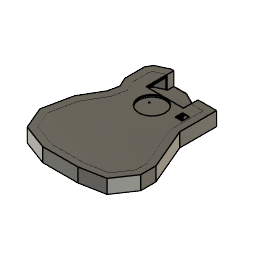
guitar body (Autodesk Fusion 360 design; units mm, degrees)
part number: 2026-05-27-12-41-13-144
Autodesk Fusion 360 part; units mm, degrees
note: some values were not read from the file. Chosen so that the rebuilt part matches the saved one: which bodies a step acts on.
sketch "Sketch1" plane through (0, 0, 0) normal (0, 0, 1) x (1, 0, 0)
  line L0 (251.1628, 0) -> (195.3488, 0)
  line L1 (195.3488, 0) -> (151.6873, -20.8028)
  line L2 (151.6873, -20.8028) -> (139.5523, -41.6057)
  line L3 (139.5523, -41.6057) -> (139.5523, -55.814)
  line L4 (139.5523, -55.814) -> (139.5523, -83.7209)
  line L5 (139.5523, -83.7209) -> (139.5523, -114.4156)
  line L6 (139.5523, -114.4156) -> (155.4368, -147.7543)
  line L7 (155.4368, -147.7543) -> (147.4945, -185.4919)
  line L8 (147.4945, -185.4919) -> (127.7472, -219.3445)
  line L9 (127.7472, -219.3445) -> (103.1629, -261.4891)
  line L10 (103.1629, -261.4891) -> (81.0774, -366.4285)
  line L11 (81.0774, -366.4285) -> (115.455, -447.2608)
  line L12 (115.455, -447.2608) -> (206.2947, -481.0654)
  line L13 (206.2947, -481.0654) -> (334.8837, -481.0654)
  line L14 (334.8837, -481.0654) -> (424.7244, -464.1631)
  line L15 (424.7244, -464.1631) -> (474.4186, -390.6977)
  line L16 (474.4186, -390.6977) -> (474.4186, -334.8837)
  line L17 (474.4186, -334.8837) -> (443.8402, -262.9846)
  line L18 (443.8402, -262.9846) -> (410.1145, -183.6851)
  line L19 (410.1145, -183.6851) -> (410.1145, -83.7209)
  line L20 (410.1145, -83.7209) -> (410.1145, -48.5399)
  line L21 (410.1145, -48.5399) -> (381.3852, -48.5399)
  line L22 (381.3852, -48.5399) -> (334.8837, -48.5399)
  line L23 (334.8837, -48.5399) -> (306.9767, -27.907)
  line L24 (306.9767, -27.907) -> (251.1628, 0)
  constraint horizontal L0
  constraint perpendicular L0 L3
  constraint perpendicular L0 L4
  constraint perpendicular L1 L6
  constraint parallel L2 L8
  constraint parallel L8 L9
  constraint parallel L7 L10
  constraint horizontal L13
  constraint vertical L16
  constraint parallel L11 L17
  constraint parallel L17 L18
  constraint parallel L16 L19
  constraint parallel L19 L20
  constraint perpendicular L20 L21
  constraint perpendicular L20 L22
extrude "Extrude1" add sketch "Sketch1" along normal blind 100 makes body 1
sketch "Sketch2" plane through (0, 0, 100) normal (0, 0, 1) x (-1, 0, 0)
  line L0 (-306.9767, 27.907) -> (-251.1628, 0)
  line L1 (-251.1628, 0) -> (-195.3488, 0)
  line L2 (-195.3488, 0) -> (-151.6873, 20.8028)
  line L3 (-151.6873, 20.8028) -> (-139.5523, 41.6057)
  line L4 (-139.5523, 41.6057) -> (-139.5523, 114.4156)
  line L5 (-139.5523, 114.4156) -> (-155.4368, 147.7543)
  line L6 (-155.4368, 147.7543) -> (-147.4945, 185.4919)
  line L7 (-147.4945, 185.4919) -> (-103.1629, 261.4891)
  line L8 (-103.1629, 261.4891) -> (-81.0774, 366.4285)
  line L9 (-81.0774, 366.4285) -> (-115.455, 447.2608)
  line L10 (-115.455, 447.2608) -> (-206.2947, 481.0654)
  line L11 (-206.2947, 481.0654) -> (-334.8837, 481.0654)
  line L12 (-334.8837, 481.0654) -> (-424.7244, 464.1631)
  line L13 (-424.7244, 464.1631) -> (-474.4186, 390.6977)
  line L14 (-474.4186, 390.6977) -> (-474.4186, 334.8837)
  line L15 (-474.4186, 334.8837) -> (-410.1145, 183.6851)
  line L16 (-410.1145, 183.6851) -> (-410.1145, 48.5399)
  line L17 (-410.1145, 48.5399) -> (-334.8837, 48.5399)
  line L18 (-334.8837, 48.5399) -> (-306.9767, 27.907)
  circle A0 centre (-275, 150) radius 48.1981
extrude "Extrude2" cut sketch "Sketch2" against normal blind 90 contours A0 bodies 1
shell "Shell1" thickness 25 removed faces 1 at (226.8618, -147.5975, 40) on bodies 1
sketch "Sketch3" plane through (0, 0, 25) normal (0, 0, 1) x (-1, 0, 0)
  circle A0 centre (-275, 150) radius 48.1981
  line L0 (-293.8574, 49.2981) -> (-245.2611, 25)
  line L1 (-245.2611, 25) -> (-201.0002, 25)
  line L2 (-201.0002, 25) -> (-169.3983, 40.0569)
  line L3 (-169.3983, 40.0569) -> (-164.5523, 48.3644)
  line L4 (-164.5523, 48.3644) -> (-164.5523, 108.7642)
  line L5 (-164.5523, 108.7642) -> (-181.6416, 144.6317)
  line L6 (-181.6416, 144.6317) -> (-171.126, 194.5966)
  line L7 (-171.126, 194.5966) -> (-126.7944, 270.5938)
  line L8 (-126.7944, 270.5938) -> (-107.1611, 363.8814)
  line L9 (-107.1611, 363.8814) -> (-134.2523, 427.581)
  line L10 (-134.2523, 427.581) -> (-210.7956, 456.0654)
  line L11 (-210.7956, 456.0654) -> (-332.5525, 456.0654)
  line L12 (-332.5525, 456.0654) -> (-409.8575, 441.5215)
  line L13 (-409.8575, 441.5215) -> (-449.4186, 383.0364)
  line L14 (-449.4186, 383.0364) -> (-449.4186, 339.9791)
  line L15 (-449.4186, 339.9791) -> (-385.1145, 188.7805)
  line L16 (-385.1145, 188.7805) -> (-385.1145, 73.5399)
  line L17 (-385.1145, 73.5399) -> (-326.6455, 73.5399)
  line L18 (-326.6455, 73.5399) -> (-293.8574, 49.2981)
extrude "Extrude3" cut sketch "Sketch3" against normal blind 20 bodies 1
sketch "Sketch4" plane through (0, 0, 100) normal (0, 0, 1) x (-1, 0, 0)
  circle A0 centre (-275, 150) radius 48.1981
  line L0 (-306.9767, 27.907) -> (-251.1628, 0)
  line L1 (-251.1628, 0) -> (-195.3488, 0)
  line L2 (-195.3488, 0) -> (-151.6873, 20.8028)
  line L3 (-151.6873, 20.8028) -> (-139.5523, 41.6057)
  line L4 (-139.5523, 41.6057) -> (-139.5523, 114.4156)
  line L5 (-139.5523, 114.4156) -> (-155.4368, 147.7543)
  line L6 (-155.4368, 147.7543) -> (-147.4945, 185.4919)
  line L7 (-147.4945, 185.4919) -> (-103.1629, 261.4891)
  line L8 (-103.1629, 261.4891) -> (-81.0774, 366.4285)
  line L9 (-81.0774, 366.4285) -> (-115.455, 447.2608)
  line L10 (-115.455, 447.2608) -> (-206.2947, 481.0654)
  line L11 (-206.2947, 481.0654) -> (-334.8837, 481.0654)
  line L12 (-334.8837, 481.0654) -> (-424.7244, 464.1631)
  line L13 (-424.7244, 464.1631) -> (-474.4186, 390.6977)
  line L14 (-474.4186, 390.6977) -> (-474.4186, 334.8837)
  line L15 (-474.4186, 334.8837) -> (-410.1145, 183.6851)
  line L16 (-410.1145, 183.6851) -> (-410.1145, 48.5399)
  line L17 (-410.1145, 48.5399) -> (-334.8837, 48.5399)
  line L18 (-334.8837, 48.5399) -> (-306.9767, 27.907)
  line L19 (-205.3595, 101.8019) -> (-341.7535, 101.8019)
  line L20 (-341.7535, 101.8019) -> (-341.7535, -17.2484)
  line L21 (-341.7535, -17.2484) -> (-205.3595, -17.2484)
  line L22 (-205.3595, -17.2484) -> (-205.3595, 101.8019)
  circle A1 centre (-335.8345, 95.8779) radius 2.3
  circle A2 centre (-211.2785, 95.8779) radius 2.3
  dimension "d9" = 136.394
  dimension "d10" = 5.919
  dimension "d11" = 5.924
  dimension "d12" = 4.6
  dimension "d13" = 5.919
  dimension "d14" = 5.924
  dimension "d15" = 4.6
  constraint horizontal L19
  constraint vertical L20
  constraint horizontal L21
  constraint vertical L22
  constraint tangent A0 L19
  measures "d9" distance of L19.start L19.end
  measures "d10" distance of L20 A1.centre
  measures "d11" distance of L19 A1.centre
  measures "d12" diameter of A1
  measures "d13" distance of L22 A2.centre
  measures "d14" distance of L19 A2.centre
  measures "d15" diameter of A2
extrude "Extrude4" cut sketch "Sketch4" against normal blind 95 contours L0 L1 L17 L18 L19 L20 L22 bodies 1 makes body 2 at (213.2984, -94.7779, 83.3333) makes body 3 at (335.102, -98.0582, 91.6667)
extrude "Extrude5" cut 1 faces at (293.8474, -161.9933, 10) along direction (0, 0, -1) blind 5 on bodies 1 bodies 1
extrude "Extrude6" cut 1 faces at (210.9984, -97.2569, 100) along direction (0, 0, -1) blind 170 on bodies 2 bodies 1 2
extrude "Extrude7" cut 1 faces at (335.6639, -96.6254, 100) along direction (0, 0, -1) blind 105 on bodies 3 bodies 1 3
extrude "Extrude8" add 1 faces at (366.8466, -337.1099, 100) along direction (0, 0, -1) blind 47.8 on bodies 1 bodies 1 2 3
extrude "Extrude9" cut 1 faces at (366.8466, -337.1099, 100) along direction (0, 0, -1) blind 40 on bodies 1 bodies 1
extrude "Extrude10" cut 1 faces at (297.4976, -283.4142, 0) along direction (0, 0, 1) blind 4 on bodies 1 bodies 1
extrude "Extrude11" add 1 faces at (355.458, -331.1055, 52.2) along direction (0, 0, -1) blind 5 separate body on bodies 1 makes body 4
extrude "Extrude12" cut 1 faces at (366.8466, -337.1099, 60) along direction (0, 0, -1) blind 5 on bodies 1 bodies 1
sketch "Sketch5" plane through (0, 0, 55) normal (0, 0, 1) x (-1, 0, 0)
  line L0 (-341.7535, 48.5399) -> (-341.7535, 101.8019)
  line L1 (-341.7535, 101.8019) -> (-275, 101.8019)
  circle A0 centre (-275, 150) radius 48.1981
  line L2 (-275, 101.8019) -> (-205.3595, 101.8019)
  line L3 (-205.3595, 101.8019) -> (-205.3595, 0)
  line L4 (-205.3595, 0) -> (-195.3489, 0)
  line L5 (-195.3489, 0) -> (-151.6873, 20.8028)
  line L6 (-151.6873, 20.8028) -> (-139.5523, 41.6057)
  line L7 (-139.5523, 41.6057) -> (-139.5523, 114.4156)
  line L8 (-139.5523, 114.4156) -> (-155.4368, 147.7543)
  line L9 (-155.4368, 147.7543) -> (-147.4946, 185.4919)
  line L10 (-147.4946, 185.4919) -> (-103.1629, 261.4891)
  line L11 (-103.1629, 261.4891) -> (-81.0774, 366.4285)
  line L12 (-81.0774, 366.4285) -> (-115.4551, 447.2608)
  line L13 (-115.4551, 447.2608) -> (-206.2947, 481.0654)
  line L14 (-206.2947, 481.0654) -> (-334.8837, 481.0654)
  line L15 (-334.8837, 481.0654) -> (-424.7245, 464.1631)
  line L16 (-424.7245, 464.1631) -> (-474.4186, 390.6977)
  line L17 (-474.4186, 390.6977) -> (-474.4186, 334.8837)
  line L18 (-474.4186, 334.8837) -> (-410.1145, 183.6851)
  line L19 (-410.1145, 183.6851) -> (-410.1145, 48.5399)
  line L20 (-410.1145, 48.5399) -> (-341.7535, 48.5399)
  line L21 (-361.3053, 120) -> (-361.3053, 142.92)
  line L22 (-361.3053, 142.92) -> (-365, 142.92)
  line L23 (-365, 142.92) -> (-365, 135)
  line L24 (-370, 135) -> (-370, 142.8017)
  line L25 (-370, 142.8017) -> (-373.9321, 142.8017)
  line L26 (-373.9321, 142.8017) -> (-373.9321, 137.5)
  line L27 (-365, 130) -> (-366.4321, 130)
  line L28 (-365, 130) -> (-365, 120)
  line L29 (-365, 120) -> (-361.3053, 120)
  arc A1 (-370, 135) -> (-365, 135) centre (-367.5, 135) ccw
  arc A2 (-373.9321, 137.5) -> (-366.4321, 130) centre (-366.4321, 137.5) ccw
  line L30 (-379.9314, 145) -> (-355, 145)
  line L31 (-355, 145) -> (-355, 118.0411)
  line L32 (-355, 118.0411) -> (-379.9314, 118.0411)
  line L33 (-379.9314, 118.0411) -> (-379.9314, 145)
  dimension "d35" = 2.5
  dimension "d36" = 7.5
  constraint perpendicular L1 L21
  constraint perpendicular L21 L22
  constraint perpendicular L1 L23
  constraint parallel L19 L24
  constraint perpendicular L24 L25
  constraint perpendicular L25 L26
  constraint horizontal L27
  constraint perpendicular L27 L28
  constraint perpendicular L21 L29
  constraint tangent L23 A1
  constraint tangent L24 A1
  constraint tangent L26 A2
  constraint tangent L27 A2
  constraint horizontal L30
  constraint vertical L31
  constraint horizontal L32
  constraint vertical L33
  measures "d35" radius of A1
  measures "d36" radius of A2
sketch "Sketch6" plane through (0, 0, 55) normal (0, 0, 1) x (-1, 0, 0)
  line L0 (-353.1908, 117.5638) -> (-382.1082, 117.5638)
  line L1 (-382.1082, 117.5638) -> (-382.1082, 147.393)
  line L2 (-382.1082, 147.393) -> (-353.1908, 147.393)
  line L3 (-353.1908, 147.393) -> (-353.1908, 117.5638)
  constraint horizontal L0
  constraint vertical L1
  constraint horizontal L2
  constraint vertical L3
extrude "Extrude13" cut sketch "Sketch5" against normal blind 2.5 contours L30 L31 L32 L33 bodies 1
sketch "Sketch7" plane through (0, 0, 5) normal (0, 0, 1) x (-1, 0, 0)
  circle A0 centre (-335.8345, 95.8779) radius 2.3
  circle A1 centre (-211.2785, 95.8779) radius 2.3
  line L0 (-205.3595, 25) -> (-201.0002, 25)
  line L1 (-201.0002, 25) -> (-169.3984, 40.0569)
  line L2 (-169.3984, 40.0569) -> (-164.5523, 48.3644)
  line L3 (-164.5523, 48.3644) -> (-164.5523, 108.7642)
  line L4 (-164.5523, 108.7642) -> (-181.6416, 144.6317)
  line L5 (-181.6416, 144.6317) -> (-171.126, 194.5966)
  line L6 (-171.126, 194.5966) -> (-126.7944, 270.5938)
  line L7 (-126.7944, 270.5938) -> (-107.1611, 363.8814)
  line L8 (-107.1611, 363.8814) -> (-134.2523, 427.581)
  line L9 (-134.2523, 427.581) -> (-210.7956, 456.0654)
  line L10 (-210.7956, 456.0654) -> (-332.5525, 456.0654)
  line L11 (-332.5525, 456.0654) -> (-409.8576, 441.5215)
  line L12 (-409.8576, 441.5215) -> (-449.4186, 383.0364)
  line L13 (-449.4186, 383.0364) -> (-449.4186, 339.9791)
  line L14 (-449.4186, 339.9791) -> (-385.1145, 188.7805)
  line L15 (-385.1145, 188.7805) -> (-385.1145, 73.5399)
  line L16 (-385.1145, 73.5399) -> (-341.7535, 73.5399)
  line L17 (-341.7535, 73.5399) -> (-341.7535, 48.5399)
  line L18 (-341.7535, 48.5399) -> (-334.8837, 48.5399)
  line L19 (-334.8837, 48.5399) -> (-306.9768, 27.907)
  line L20 (-306.9768, 27.907) -> (-251.1628, 0)
  line L21 (-251.1628, 0) -> (-205.3595, 0)
  line L22 (-205.3595, 0) -> (-205.3595, 25)
  line L23 (-200, 387.3021) -> (-378.0045, 387.3021) construction
  line L24 (-378.0045, 387.3021) -> (-378.0045, 325) construction
  line L25 (-378.0045, 325) -> (-200, 325) construction
  line L26 (-200, 325) -> (-200, 387.3021) construction
  dimension "d39" = 10
sketch "Sketch8" plane through (0, 0, 4) normal (0, 0, -1) x (1, 0, 0)
  circle A0 centre (335.8345, 95.8779) radius 2.3
  circle A1 centre (211.2785, 95.8779) radius 2.3
  line L0 (251.1628, 0) -> (306.9768, 27.907)
  line L1 (306.9768, 27.907) -> (334.8837, 48.5399)
  line L2 (334.8837, 48.5399) -> (410.1145, 48.5399)
  line L3 (410.1145, 48.5399) -> (410.1145, 183.6851)
  line L4 (410.1145, 183.6851) -> (474.4186, 334.8837)
  line L5 (474.4186, 334.8837) -> (474.4186, 390.6977)
  line L6 (474.4186, 390.6977) -> (424.7245, 464.1631)
  line L7 (424.7245, 464.1631) -> (334.8837, 481.0654)
  line L8 (334.8837, 481.0654) -> (206.2947, 481.0654)
  line L9 (206.2947, 481.0654) -> (115.4551, 447.2608)
  line L10 (115.4551, 447.2608) -> (81.0774, 366.4285)
  line L11 (81.0774, 366.4285) -> (103.1629, 261.4891)
  line L12 (103.1629, 261.4891) -> (147.4946, 185.4919)
  line L13 (147.4946, 185.4919) -> (155.4368, 147.7543)
  line L14 (155.4368, 147.7543) -> (139.5523, 114.4156)
  line L15 (139.5523, 114.4156) -> (139.5523, 41.6057)
  line L16 (139.5523, 41.6057) -> (151.6873, 20.8028)
  line L17 (151.6873, 20.8028) -> (195.3489, 0)
  line L18 (195.3489, 0) -> (251.1628, 0)
  line L19 (400, 400) -> (350, 400) construction
  line L20 (350, 400) -> (350, 380) construction
  line L21 (350, 380) -> (400, 380) construction
  line L22 (400, 380) -> (400, 400) construction
  dimension "d41" = 10
  text T0 "chrifko" font "Arial" height 10 align left top in box 50 x 20 at (400, 400) x (-1, 0) y (0, -1) spacing 1
extrude "Extrude14" cut sketch "Sketch8" against normal blind 1 text T0 bodies 1 makes body 5 at (363.7802, -384.5437, 4)
equation "d40 = 'chrifko'"
equation "d42 = 'chrifko'"
